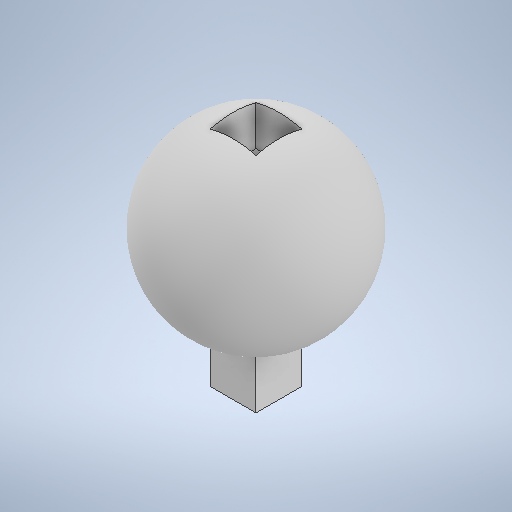
# Autodesk Inventor part: CVTag
Saved by Autodesk Inventor 2025.2 (Build 292293000, 293)
## iProperties
Created: 2025-03-26
Part Number: CVTag
Material: Generic
Document SubType Name: Modeling
Designer: Marcu
Density: 1 g/cm^3
Appearance: Default
Author: Marcu
Autodesk Inventor part; units mm, degrees
ref_plane "YZ Plane" through (0, 0, 0) normal (1, 0, 0) x (0, 1, 0)
ref_plane "XZ Plane" through (0, 0, 0) normal (0, 1, 0) x (-1, 0, 0)
ref_plane "XY Plane" through (0, 0, 0) normal (0, 0, 1) x (1, 0, 0)
sketch "Sketch1" plane through (0, 0, 0) normal (0, 1, 0) x (-1, 0, 0)
  line L0 (-2.5, -2.5) -> (2.5, -2.5)
  line L1 (2.5, -2.5) -> (2.5, 2.5)
  line L2 (2.5, 2.5) -> (-2.5, 2.5)
  line L3 (-2.5, 2.5) -> (-2.5, -2.5)
  point P0 (0, 0)
  dimension "d0" = 2.5
  dimension "d1" = 2.5
  dimension "d2" = 5
  dimension "d3" = 5
  constraints: 8 end point, 2 parallel, 1 horizontal, 1 perpendicular
  measures "d0" distance from line of point (0, 0) L2
  measures "d1" distance from line of point (0, 0) L1
  measures "d2" distance between parallel lines of L2 L0
  measures "d3" distance between parallel lines of L3 L1
extrude "Extrusion1" add sketch "Sketch1" along normal blind 15
sketch "Sketch2" plane through (0, 0, 0) normal (0, 0, 1) x (1, 0, 0)
  line L0 (-2.5, 15) -> (2.5, 15) projected
  arc A0 (0, 25) -> (0, 5) centre (0, 15) ccw
  line L1 (0, 25) -> (0, 5)
  point P0 (0, 0)
  constraints: 2 end point, 2 midpoint, 2 point on circle, 1 centre point, 1 vertical
revolve "Revolution1" add sketch "Sketch2" angle 360 about axis through (0, 25, 0) along (0, -1, 0)
sketch "Sketch3" plane through (0, 0, 0) normal (0, 0, 1) x (1, 0, 0)
  line L0 (2.5, 25) -> (-2.5, 25)
  line L1 (-2.5, 25) -> (-2.5, 20)
  line L2 (-2.5, 20) -> (2.5, 20)
  line L3 (2.5, 20) -> (2.5, 25)
  point P0 (0, 0)
  dimension "d8" = 2.5
  dimension "d9" = 5
  dimension "d10" = 5
  dimension "d11" = 25
  constraints: 8 end point, 2 parallel, 1 horizontal, 1 perpendicular
  measures "d8" distance from line of point (0, 0) L3
  measures "d9" distance between parallel lines of L3 L1
  measures "d10" distance between parallel lines of L2 L0
  measures "d11" distance from line of point (0, 0) L0
extrude "Extrusion2" cut sketch "Sketch3" along normal mid plane 5
body "Solid1"
